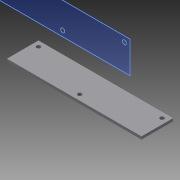
# Autodesk Inventor part: konektor kort
Saved by Autodesk Inventor 2015 (Build 190159000, 159)
## iProperties
Created: 2015-08-04
Part Number: konektor kort
Material: Generic
Document SubType Name: Modeling
Designer: Simen
Density: 1 g/cm^3
Appearance: Default
Author: Simen
Autodesk Inventor part; units mm, degrees
ref_plane "YZ Plane" through (0, 0, 0) normal (1, 0, 0) x (0, 1, 0)
ref_plane "XZ Plane" through (0, 0, 0) normal (0, 1, 0) x (-1, 0, 0)
ref_plane "XY Plane" through (0, 0, 0) normal (0, 0, 1) x (1, 0, 0)
sketch "Sketch1" plane through (0, 0, 0) normal (0, 0, 1) x (1, 0, 0)
  line L0 (27.1862, 25.2035) -> (-70.8138, 25.2035)
  line L1 (-70.8138, 25.2035) -> (-70.8138, 2.2035)
  line L2 (-70.8138, 2.2035) -> (27.1862, 2.2035)
  line L3 (27.1862, 2.2035) -> (27.1862, 25.2035)
  line L4 (27.1862, 25.2035) -> (27.1862, 21.2035)
  line L5 (27.1862, 21.2035) -> (23.1862, 21.2035)
  circle A0 centre (23.1862, 21.2035) radius 1.5
  line L6 (-70.8138, 25.2035) -> (-70.8138, 21.2035)
  line L7 (-70.8138, 21.2035) -> (-66.8138, 21.2035)
  circle A1 centre (-66.8138, 21.2035) radius 1.5
  line L8 (-21.8138, 2.2035) -> (-21.8138, 6.2035)
  circle A2 centre (-21.8138, 6.2035) radius 1.5
  point P0 (0, 0)
  dimension "d0" = 98
  dimension "d1" = 23
  dimension "d2" = 4
  dimension "d3" = 4
  dimension "d4" = 3
  dimension "d5" = 4
  dimension "d6" = 4
  dimension "d7" = 3
  dimension "d8" = 4
  dimension "d9" = 3
  constraints: 18 end point, 3 centre point, 3 coincident, 3 perpendicular, 2 parallel, 2 point on line, 1 horizontal, 1 midpoint, 1 vertical
  measures "d0" distance of L2.end L1.end
  measures "d1" distance of L1.end L0.end
  measures "d2" distance of L0.start L4.end
  measures "d3" distance of L4.end L5.end
  measures "d4" diameter of A0
  measures "d5" distance of L0.end L6.end
  measures "d6" distance of L6.end L7.end
  measures "d7" diameter of A1
  measures "d8" distance of L8.start L8.end
  measures "d9" diameter of A2
extrude "Extrusion1" add sketch "Sketch1" along normal blind 2
body "Solid1"
